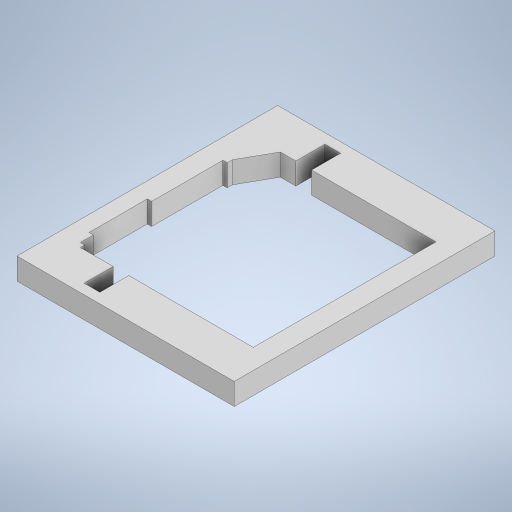
# Autodesk Inventor part: OMG_20kg_servo_side_profile(0.4mm)
Saved by Autodesk Inventor 2023.1 (Build 271208000, 208)
## iProperties
Created: 2026-02-21
Part Number: OMG_20kg_servo_side_profile(0.4mm)
Material: Generic
Document SubType Name: Modeling
Designer: Lars
Density: 1 g/cm^3
Appearance: Default
Author: Lars
Autodesk Inventor part; units mm, degrees
ref_plane "YZ Plane" through (0, 0, 0) normal (1, 0, 0) x (0, 1, 0)
ref_plane "XZ Plane" through (0, 0, 0) normal (0, 1, 0) x (-1, 0, 0)
ref_plane "XY Plane" through (0, 0, 0) normal (0, 0, 1) x (1, 0, 0)
sketch "Sketch1" plane through (0, 0, 0) normal (0, 1, 0) x (-1, 0, 0)
  line L0 (0, 0) -> (28.63, 0)
  line L1 (28.63, 0) -> (28.63, -41.25) construction
  line L2 (28.63, -41.25) -> (0, -41.25)
  line L3 (0, -41.25) -> (0, 0)
  line L4 (28.63, 6.675) -> (31.43, 6.675)
  line L5 (31.43, 6.675) -> (31.43, 0)
  line L6 (31.43, -47.925) -> (28.63, -47.925)
  line L7 (28.63, -47.925) -> (28.63, -41.25)
  line L8 (31.43, -20.625) -> (28.63, -20.625) construction
  line L9 (38.98, 0) -> (31.43, 0)
  line L10 (31.43, 0) -> (31.43, -41.25) construction
  line L11 (31.43, -41.25) -> (35.18, -41.25)
  line L12 (38.98, -41.25) -> (38.98, -34.5) construction
  line L13 (31.43, -41.25) -> (35.18, -41.25) construction
  line L14 (38.98, 0) -> (38.98, -1) construction
  line L15 (38.98, -34.5) -> (35.18, -41.25)
  line L16 (38.98, -34.5) -> (38.98, -33)
  line L17 (35.18, -41.25) -> (38.98, -41.25) construction
  line L18 (38.98, 0) -> (38.98, -1) construction
  line L19 (38.98, -1) -> (39.98, -1)
  line L20 (39.98, -1) -> (39.98, -4)
  line L21 (39.98, -33) -> (38.98, -33)
  line L22 (38.98, -33) -> (38.98, -1) construction
  line L23 (38.98, -1) -> (38.98, -33) construction
  line L24 (38.98, -33) -> (38.98, -34.5) construction
  line L25 (38.98, -1) -> (38.98, 0)
  line L26 (38.98, -33) -> (38.98, -1) construction
  line L27 (31.43, 0) -> (31.43, -41.25) construction
  line L28 (31.43, -41.25) -> (31.43, -47.925)
  line L29 (28.63, -41.25) -> (28.63, 0) construction
  line L30 (28.63, 0) -> (28.63, 6.675)
  line L31 (28.63, 0) -> (31.43, 0) construction
  line L32 (31.43, -41.25) -> (28.63, -41.25) construction
  line L33 (39.98, -1) -> (39.98, -4) construction
  line L34 (39.98, -4) -> (40.98, -4)
  line L35 (40.98, -4) -> (40.98, -16.6)
  line L36 (40.98, -16.6) -> (39.98, -16.6)
  line L37 (39.98, -16.6) -> (39.98, -4) construction
  line L38 (39.98, -4) -> (39.98, -16.6) construction
  line L39 (39.98, -16.6) -> (39.98, -33)
  line L40 (41.38, -17) -> (41.38, -3.6)
  line L41 (41.38, -3.6) -> (40.38, -3.6)
  line L42 (40.38, -3.6) -> (40.38, -0.6)
  line L43 (40.38, -0.6) -> (39.38, -0.6)
  line L44 (39.38, -0.6) -> (39.38, 0.4)
  line L45 (39.38, 0.4) -> (31.83, 0.4)
  line L46 (31.83, 0.4) -> (31.83, 7.075)
  line L47 (31.83, 7.075) -> (28.23, 7.075)
  line L48 (28.23, 7.075) -> (28.23, 0.4)
  line L49 (28.23, 0.4) -> (-0.4, 0.4)
  line L50 (-0.4, 0.4) -> (-0.4, -41.65)
  line L51 (-0.4, -41.65) -> (28.23, -41.65)
  line L52 (28.23, -41.65) -> (28.23, -48.325)
  line L53 (28.23, -48.325) -> (31.83, -48.325)
  line L54 (31.83, -48.325) -> (31.83, -41.65)
  line L55 (31.83, -41.65) -> (35.4138, -41.65)
  line L56 (35.4138, -41.65) -> (39.38, -34.6049)
  line L57 (39.38, -34.6049) -> (39.38, -33.4)
  line L58 (39.38, -33.4) -> (40.38, -33.4)
  line L59 (40.38, -33.4) -> (40.38, -17)
  line L60 (40.38, -17) -> (41.38, -17)
  line L61 (0, -20.625) -> (39.98, -20.625) construction
  line L62 (44.99, 9.375) -> (-5.01, 9.375)
  line L63 (-5.01, 9.375) -> (-5.01, -50.625)
  line L64 (-5.01, -50.625) -> (44.99, -50.625)
  line L65 (44.99, -50.625) -> (44.99, 9.375)
  line L66 (19.99, 9.375) -> (19.99, -50.625) construction
  point P0 (30.03, 6.675)
  point P1 (19.99, -20.625)
  dimension "d0" = 28.63
  dimension "d1" = 41.25
  dimension "d2" = 2.8
  dimension "d3" = 54.6
  dimension "d4" = 7.55
  dimension "d5" = 41.25
  dimension "d6" = 3.75
  dimension "d7" = 34.5
  dimension "d8" = 1
  dimension "d9" = 32
  dimension "d10" = 1
  dimension "d11" = 6.675
  dimension "d12" = 3
  dimension "d13" = 1
  dimension "d14" = 12.6
  dimension "d15" = 0.4
  dimension "d16" = 50
  dimension "d17" = 60
  constraints: 134 end point, 35 parallel, 17 perpendicular, 8 midpoint, 7 horizontal, 5 vertical, 1 point on line, 20 other
  measures "d0" distance of L1.end L2.end
  measures "d1" distance of L0.end L1.end
  measures "d2" distance of L6.start L6.end
  measures "d3" distance of L4.end L6.start
  measures "d4" distance of L12.start L10.end
  measures "d5" distance of L12.start L9.start
  measures "d6" distance of L10.end L11.end
  measures "d7" distance of L9.start L12.end
  measures "d8" distance of L9.start L14.end
  measures "d9" distance of L19.end L21.start
  measures "d10" distance of L21.start L16.end
  measures "d11" distance from line of point (30.03, 6.675) L31
  measures "d12" distance of L19.end L20.end
  measures "d13" distance of L35.end L36.end
  measures "d14" distance of L34.end L35.end
  measures "d15" distance between parallel lines of L35 L40
  measures "d16" distance of L64.end L63.end
  measures "d17" distance of L63.end L62.end
extrude "Extrusion1" add sketch "Sketch1" along normal blind 5 contours L65 L64 L63 L62
equation "\"d5\" = d1"
body "Solid1"
